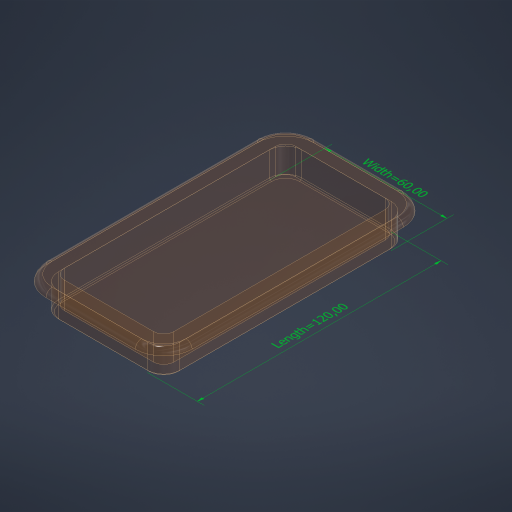
# Autodesk Inventor part: Holder
Saved by Autodesk Inventor 2024.3 (Build 283343000, 343)
## iProperties
Company: UAB Čeli APS
Created: 2022-04-25
Part Number: Holder
Material: Polycarbonate, Smoke
Document SubType Name: Modeling
Designer: sauliusd
Density: 1.2 g/cm^3
Appearance: Polycarbonate - Smoked
Description: Holder for paper clips.ipt
Width: 60,000 mm
Length: 120,000 mm
Author: S. Dereškevičius
Autodesk Inventor part; units mm, degrees
ref_plane "YZ Plane" through (0, 0, 0) normal (1, 0, 0) x (0, 1, 0)
ref_plane "XZ Plane" through (0, 0, 0) normal (0, 1, 0) x (-1, 0, 0)
ref_plane "XY Plane" through (0, 0, 0) normal (0, 0, 1) x (1, 0, 0)
sketch "Sketch1" plane through (0, 0, 0) normal (0, 0, 1) x (1, 0, 0)
  line L0 (-60, -30) -> (60, -30)
  line L1 (60, -30) -> (60, 30)
  line L2 (60, 30) -> (-60, 30)
  line L3 (-60, 30) -> (-60, -30)
  line L4 (-60, -30) -> (60, 30) construction
  line L5 (60, -30) -> (-60, 30) construction
  point P0 (0, 0)
  constraints: 12 end point, 2 midpoint, 2 parallel, 1 horizontal, 1 horizontal alignment, 1 perpendicular, 1 vertical alignment
extrude "Extrusion1" add sketch "Sketch1" along normal blind 13
fillet "Fillet1" radius 8 4 edges at (-60, -30, 6.5) (-60, 30, 6.5) (60, -30, 6.5) (60, 30, 6.5)
shell "Shell1" thickness 3 removed faces 1 at (17.3333, -10, 13)
sketch "Sketch2" plane through (0, 0, 13) normal (0, 0, 1) x (1, 0, 0)
  arc A0 (60, 22) -> (52, 30) centre (52, 22) ccw projected
  line L0 (52, 30) -> (-52, 30) projected
  arc A1 (-52, 30) -> (-60, 22) centre (-52, 22) ccw projected
  line L1 (-60, 22) -> (-60, -22) projected
  arc A2 (-60, -22) -> (-52, -30) centre (-52, -22) ccw projected
  line L2 (-52, -30) -> (52, -30) projected
  arc A3 (52, -30) -> (60, -22) centre (52, -22) ccw projected
  line L3 (60, -22) -> (60, 22) projected
  line L4 (-52, 36) -> (52, 36)
  arc A4 (66, 22) -> (52, 36) centre (52, 22) ccw
  line L5 (66, 22) -> (66, -22)
  arc A5 (52, -36) -> (66, -22) centre (52, -22) ccw
  line L6 (52, -36) -> (-52, -36)
  arc A6 (-66, -22) -> (-52, -36) centre (-52, -22) ccw
  line L7 (-66, -22) -> (-66, 22)
  arc A7 (-52, 36) -> (-66, 22) centre (-52, 22) ccw
  arc A8 (-52, 27) -> (-57, 22) centre (-52, 22) ccw projected
  line L8 (-52, 27) -> (52, 27) projected
  arc A9 (57, 22) -> (52, 27) centre (52, 22) ccw projected
  line L9 (57, 22) -> (57, -22) projected
  arc A10 (52, -27) -> (57, -22) centre (52, -22) ccw projected
  line L10 (52, -27) -> (-52, -27) projected
  arc A11 (-57, -22) -> (-52, -27) centre (-52, -22) ccw projected
  line L11 (-57, -22) -> (-57, 22) projected
  arc A12 (60, 22) -> (52, 30) centre (52, 22) ccw projected
  line L12 (52, 30) -> (-52, 30) projected
  arc A13 (-52, 30) -> (-60, 22) centre (-52, 22) ccw projected
  line L13 (-60, 22) -> (-60, -22) projected
  arc A14 (-60, -22) -> (-52, -30) centre (-52, -22) ccw projected
  line L14 (-52, -30) -> (52, -30) projected
  arc A15 (52, -30) -> (60, -22) centre (52, -22) ccw projected
  line L15 (60, -22) -> (60, 22) projected
  point P0 (0, 0)
  dimension "d5" = 6
  constraints: 8 end point, 8 point on circle, 4 centre point, 7 other
  measures "d5" distance between parallel lines of L0 L4
extrude "Extrusion2" add sketch "Sketch2" along normal blind 3 contours L3 A3 L2 A2 L1 A1 L0 A0 | L4 A4 L5 A5 L6 A6 L7 A7
fillet "Fillet2" radius 3 8 edges at (-66, 0, 16) (-61.8995, -31.8995, 16) (0, -36, 16) (61.8995, -31.8995, 16) (66, 0, 16) (61.8995, 31.8995, 16) (0, 36, 16) (-61.8995, 31.8995, 16)
sketch "Sketch3" plane through (0, 0, 0) normal (0, 0, -1) x (-1, 0, 0)
  arc A0 (-52, 30) -> (-60, 22) centre (-52, 22) ccw projected
  line L0 (-60, -22) -> (-60, 22) projected
  arc A1 (-60, -22) -> (-52, -30) centre (-52, -22) ccw projected
  line L1 (52, -30) -> (-52, -30) projected
  arc A2 (52, -30) -> (60, -22) centre (52, -22) ccw projected
  line L2 (60, 22) -> (60, -22) projected
  arc A3 (60, 22) -> (52, 30) centre (52, 22) ccw projected
  line L3 (-52, 30) -> (52, 30) projected
  point P0 (0, 0)
chamfer "Chamfer1" distance 1 angle 45 8 edges at (-60, 0, 0) (-57.6569, -27.6569, 0) (0, -30, 0) (57.6569, -27.6569, 0) (60, 0, 0) (57.6569, 27.6569, 0) (0, 30, 0) (-57.6569, 27.6569, 0)
extrude "Extrusion3" add sketch "Sketch3" against normal up to surface (13 mm away) separate body
sketch "Sketch4" plane through (-52, 30, 13) normal (0, 0, 1) x (1, 0, 0)
  line L0 (112, -8) -> (112, -52) projected
  line L1 (0, 0) -> (104, 0) projected
  point P0 (52, -30)
  point P1 (112, -30)
  point P2 (52, 0)
  constraints: 2 midpoint
equation "\"zzz\" = 1"
